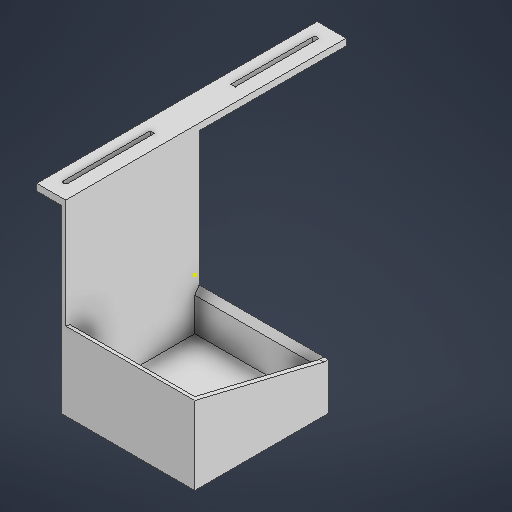
# Autodesk Inventor part: pickup_cup
Saved by Autodesk Inventor 2026.1 (Build 301233020, 233B)
## iProperties
Created: 2025-12-16
Part Number: pickup_cup
Material: Generic
Document SubType Name: Modeling
Designer: andmi
Density: 1 g/cm^3
Appearance: Default
Author: andmi
Autodesk Inventor part; units mm, degrees
ref_plane "YZ Plane" through (0, 0, 0) normal (1, 0, 0) x (0, 1, 0)
ref_plane "XZ Plane" through (0, 0, 0) normal (0, 1, 0) x (-1, 0, 0)
ref_plane "XY Plane" through (0, 0, 0) normal (0, 0, 1) x (1, 0, 0)
sketch "Sketch1" plane through (0, 0, 0) normal (0, 1, 0) x (-1, 0, 0)
  line L0 (0, 0) -> (60, 0)
  line L1 (60, 0) -> (60, -60)
  line L2 (60, -60) -> (0, -60)
  line L3 (0, -60) -> (0, 0)
  dimension "d0" = 60
  dimension "d1" = 60
  constraints: 8 end point, 2 parallel, 1 horizontal, 1 perpendicular
  measures "d0" distance of L0.end L1.end
  measures "d1" distance of L1.end L2.end
extrude "Extrusion1" add sketch "Sketch1" along normal blind 3
sketch "Sketch3" plane through (0, 3, 0) normal (0, 1, 0) x (1, 0, 0)
  line L0 (0, 60) -> (-60, 60) projected
  line L1 (0, 0) -> (0, 60) projected
  line L2 (-60, 60) -> (0, 60)
  line L3 (0, 60) -> (0, 58)
  line L4 (0, 58) -> (-60, 58)
  line L5 (-60, 58) -> (-60, 60)
  dimension "d4" = 2
  constraints: 8 end point, 2 parallel, 1 horizontal, 1 perpendicular, 1 point on line
  measures "d4" distance of L4.end L0.end
extrude "Extrusion2" add sketch "Sketch3" along normal blind 18
sketch "Sketch4" plane through (0, 0, 0) normal (1, 0, 0) x (0, 0, -1)
  line L0 (0, 3) -> (58, 3) projected
  line L1 (0, 3) -> (0, 35)
  line L2 (60, 21) -> (58, 21) projected
  line L3 (0, 35) -> (58, 21)
  line L4 (58, 21) -> (58, 3)
  line L5 (58, 3) -> (0, 3)
  point P0 (0, 0)
  dimension "d7" = 32
  constraints: 8 end point, 1 parallel, 1 perpendicular, 1 vertical
  measures "d7" distance of L0.start L1.end
extrude "Extrusion3" add sketch "Sketch4" against normal blind 2
sketch "Sketch5" plane through (-60, 0, -60) normal (-1, 0, 0) x (0, 0, 1)
  line L0 (2, 21) -> (0, 21) projected
  line L1 (0, 21) -> (2, 18)
  line L2 (2, 3) -> (2, 21) projected
  line L3 (2, 18) -> (2, 21)
  line L4 (2, 21) -> (0, 21)
  line L5 (0, 0) -> (0, 21) projected
  point P0 (60, 0)
  dimension "d10" = 3
  constraints: 6 end point, 3 point on line, 1 vertical
  measures "d10" distance of L0.start L1.end
extrude "Extrusion4" cut sketch "Sketch5" against normal blind 58
sketch "Sketch6" plane through (-60, 0, -60) normal (-1, 0, 0) x (0, 0, 1)
  line L0 (0, 0) -> (0, 21) projected
  line L1 (0, 21) -> (2, 21)
  line L2 (60, 35) -> (2, 21) projected
  line L3 (2, 21) -> (60, 35)
  line L4 (60, 35) -> (60, 0)
  line L5 (60, 0) -> (0, 0) projected
  line L6 (60, 0) -> (0, 0)
  line L7 (0, 0) -> (0, 21)
  constraints: 10 end point, 2 collinear, 2 perpendicular
extrude "Extrusion5" add sketch "Sketch6" against normal blind 2
sketch "Sketch8" plane through (-58, 0, -60) normal (1, 0, 0) x (0, 0, -1)
  line L0 (-2, 3) -> (-60, 3) projected
  line L1 (-60, 3) -> (-58, 3)
  line L2 (-58, 3) -> (-58, 34.5172)
  line L3 (-2, 21) -> (-60, 35) projected
  line L4 (-58, 34.5172) -> (-60, 35)
  line L5 (-60, 35) -> (-60, 3)
  point P0 (-60, 0)
  dimension "d15" = 2
  constraints: 8 end point, 2 point on line, 1 collinear, 1 parallel, 1 perpendicular
  measures "d15" distance between parallel lines of L2 L5
extrude "Extrusion6" add sketch "Sketch8" along normal blind 56
sketch "Sketch9" plane through (-60, 0, -60) normal (-1, 0, 0) x (0, 0, 1)
  line L0 (0, 21) -> (2, 21) projected
  line L1 (0, 21) -> (60, 21)
  line L2 (60, 21) -> (60, 81)
  line L3 (60, 81) -> (0, 81)
  line L4 (0, 81) -> (0, 21)
  point P0 (60, 0)
  dimension "d18" = 60
  dimension "d19" = 60
  constraints: 8 end point, 2 parallel, 1 horizontal, 1 perpendicular
  measures "d18" distance of L2.end L3.end
  measures "d19" distance of L1.end L2.end
extrude "Extrusion7" add sketch "Sketch9" against normal blind 2
sketch "Sketch11" plane through (-58, 0, -60) normal (1, 0, 0) x (0, 0, -1)
  line L0 (0, 81) -> (-60, 81) projected
  line L1 (-60, 81) -> (66, 81)
  line L2 (66, 81) -> (66, 84)
  line L3 (66, 84) -> (-60, 84)
  line L4 (-60, 84) -> (-60, 81)
  point P0 (-60, 0)
  dimension "d26" = 3
  dimension "d27" = 126
  constraints: 8 end point, 2 parallel, 1 horizontal, 1 perpendicular
  measures "d26" distance of L3.end L0.end
  measures "d27" distance of L2.end L3.end
extrude "Extrusion9" add sketch "Sketch11" against normal blind 13
sketch "Sketch12" plane through (-58, 84, 0) normal (0, 1, 0) x (1, 0, 0)
  circle A0 centre (-7, 119) radius 1
  line L0 (0, 126) -> (-13, 126) projected
  line L1 (0, 126) -> (0, 0) projected
  circle A1 centre (-7, 7) radius 1
  line L2 (0, 0) -> (-13, 0) projected
  point P0 (58, 0)
  dimension "d30" = 2
  dimension "d31" = 7
  dimension "d32" = 7
  dimension "d33" = 2
  dimension "d34" = 7
  dimension "d35" = 7
  constraints: 2 centre point
  measures "d30" diameter of A0
  measures "d31" distance from line of L0 A0.centre
  measures "d32" distance from line of A0.centre L1
  measures "d33" diameter of A1
  measures "d34" distance from line of L2 A1.centre
  measures "d35" distance from line of A1.centre L1
extrude "Extrusion10" cut sketch "Sketch12" against normal blind 13
sketch "Sketch13" plane through (-58, 84, 0) normal (0, 1, 0) x (1, 0, 0)
  circle A0 centre (-7, 7) radius 1 projected
  line L0 (-8, 7) -> (-8, 119)
  line L1 (-8, 119) -> (-6, 119)
  line L2 (-6, 119) -> (-6, 7)
  line L3 (-6, 7) -> (-8, 7)
  circle A1 centre (-7, 119) radius 1 projected
  point P0 (58, 0)
  dimension "d40" = 0
  constraints: 8 end point, 2 point on circle, 2 tangent, 1 horizontal, 1 perpendicular, 1 vertical
  measures "d40" distance from line of L1 A1.centre
extrude "Extrusion11" cut sketch "Sketch13" against normal blind 10 contours A0 L0 A1 L2 | A1 L1 picked at (-6.9598, 118.6691)
sketch "Sketch14" plane through (-58, 84, 0) normal (0, 1, 0) x (1, 0, 0)
  point P0 (58, 0)
sketch "Sketch15" plane through (-58, 84, 0) normal (0, 1, 0) x (1, 0, 0)
  line L0 (-11.1798, 45.8772) -> (-2.4734, 45.8772)
  line L1 (-2.4734, 45.8772) -> (-2.4734, 82.1146)
  line L2 (-2.4734, 82.1146) -> (-11.1798, 82.1146)
  line L3 (-11.1798, 82.1146) -> (-11.1798, 45.8772)
  point P0 (58, 0)
  constraints: 8 end point, 2 parallel, 1 horizontal, 1 perpendicular
extrude "Extrusion12" add sketch "Sketch15" against normal blind 3
body "Solid1"
